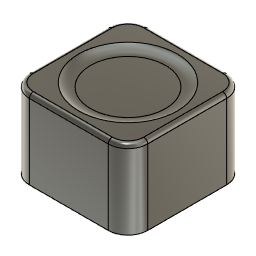
reset keys v2 (Autodesk Fusion 360 design; units mm, degrees)
Autodesk Fusion 360 part; units mm, degrees
sketch "Sketch1" plane through (0, 0, 0) normal (0, 0, 1) x (1, 0, 0)
  line L0 (3, -3) -> (-3, -3)
  line L1 (-3, -3) -> (-3, 3)
  line L2 (-3, 3) -> (3, 3)
  line L3 (3, 3) -> (3, -3)
  line L4 (3, -3) -> (-3, 3) construction
  line L5 (-3, -3) -> (3, 3) construction
  dimension "d1" = 6
  dimension "d2" = 6
  constraint horizontal L0
  constraint perpendicular L0 L1
  constraint parallel L0 L2
  constraint parallel L1 L3
  constraint coincident L4 origin
  constraint coincident L5 origin
  measures "d1" distance of L1.end L2.end
  measures "d2" distance of L0.end L1.end
extrude "Extrude1" add sketch "Sketch1" along normal blind 4
sketch "Sketch2" plane through (0, 0, 4) normal (0, 0, 1) x (-1, 0, 0)
  line L0 (-3, -3) -> (3, -3)
  line L1 (3, -3) -> (3, 3)
  line L2 (3, 3) -> (-3, 3)
  line L3 (-3, 3) -> (-3, -3)
  circle A0 centre (0, 0) radius 2.5
  dimension "d7" = 5
  constraint coincident A0.centre origin
  measures "d7" diameter of A0
extrude "Extrude2" cut sketch "Sketch2" against normal blind 0.2 contours A0
fillet "Fillet1" radius 1 1 edges at (2.3308, -0.904, 3.8)
fillet "Fillet2" radius 0.2 4 edges at (-3, 0, 4) (0, 3, 4) (3, 0, 4) (0, -3, 4)
fillet "Fillet3" radius 1 8 edges at (3, -3, 1.9) (2.9414, -2.9414, 3.9414) (-3, -3, 1.9) (-2.9414, -2.9414, 3.9414) (3, 3, 1.9) (2.9414, 2.9414, 3.9414) (-3, 3, 1.9) (-2.9414, 2.9414, 3.9414)
equation "d2 = d1"
